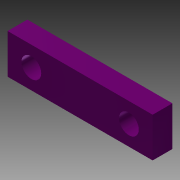
# Autodesk Inventor part: 知能ロボコン砲身止め
Saved by Autodesk Inventor 2013 (Build 170138000, 138)
## iProperties
Created: 2014-08-21
Part Number: 知能ロボコン砲身止め
Material: ABS プラスチック
Document SubType Name: Modeling
Designer: horumo136
Density: 1 g/cm^3
Author: horumo136
Autodesk Inventor part; units mm, degrees
ref_plane "YZ Plane" through (0, 0, 0) normal (1, 0, 0) x (0, 1, 0)
ref_plane "XZ Plane" through (0, 0, 0) normal (0, 1, 0) x (-1, 0, 0)
ref_plane "XY Plane" through (0, 0, 0) normal (0, 0, 1) x (1, 0, 0)
sketch "スケッチ1" plane through (0, 0, 0) normal (0, 1, 0) x (-1, 0, 0)
  line L0 (0, 0) -> (-14.8, 0)
  circle A0 centre (-14.8, 0) radius 1.5
  circle A1 centre (0, 0) radius 1.5
  line L1 (-18.4, 3) -> (3.6, 3)
  line L2 (3.6, 3) -> (3.6, -3)
  line L3 (3.6, -3) -> (-18.4, -3)
  line L4 (-18.4, -3) -> (-18.4, 3)
  line L5 (-18.4, 3) -> (3.6, -3) construction
  line L6 (3.6, 3) -> (-18.4, -3) construction
  point P0 (-7.4, 0)
  dimension "d0" = 14.8
  dimension "d1" = 3
  dimension "d2" = 3
  dimension "d3" = 22
  dimension "d4" = 6
  constraints: 14 end point, 3 midpoint, 2 centre point, 2 coincident, 2 horizontal, 2 parallel, 1 perpendicular
  measures "d0" distance of L0.start L0.end
  measures "d1" diameter of A0
  measures "d2" diameter of A1
  measures "d3" distance of L2.end L3.end
  measures "d4" distance of L1.end L2.end
extrude "押し出し1" add sketch "スケッチ1" along normal blind 3
